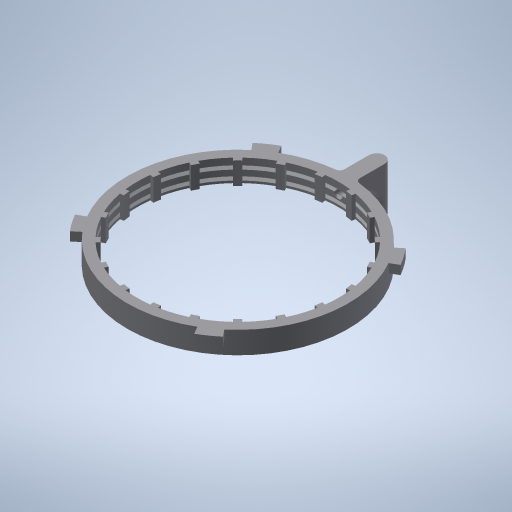
# Autodesk Inventor part: Sealing_ring_20x1_silicone_i
Saved by Autodesk Inventor 2023.2 (Build 272271000, 271)
## iProperties
Created: 2022-11-16
Part Number: Sealing_ring_20x1_silicone_i
Material: Generisch
Document SubType Name: Modeling
Designer: splath
Density: 1 g/cm^3
Appearance: Vorgabe
Author: splath
Autodesk Inventor part; units mm, degrees
ref_plane "Work Plane3" through (0, 0, 4) normal (0, 0, -1) x (0, -1, 0)
ref_plane "YZ Plane" through (0, 0, 0) normal (1, 0, 0) x (0, 1, 0)
sketch "Sketch1" plane through (0, 0, 0) normal (0, 1, 0) x (-1, 0, 0)
  line L0 (20.5, 5.8) -> (20.5, 4.7008) construction
  line L1 (22, 0) -> (25, 0)
  line L2 (25, 0) -> (25, 5)
  line L3 (25, 5) -> (22.8, 5)
  line L4 (21.5, 5) -> (21.5, 5.8) construction
  line L5 (21.5, 5.8) -> (20.5, 5.8) construction
  line L6 (0, -10.2759) -> (0, 12.2292) construction
  line L7 (30, 0) -> (-5, 0) construction
  line L8 (0, 9.0142) -> (16.75, 9.0142) construction
  line L9 (16.75, 9.0142) -> (16.75, -7.0609) construction
  line L10 (16.75, -7.0609) -> (0, -7.0609) construction
  line L11 (0, -7.0609) -> (0, 9.0142) construction
  line L12 (22, 0.2899) -> (22, 0)
  line L13 (23.3, 2.0523) -> (24.0071, 1.3452)
  line L14 (24.0071, 1.3452) -> (22.5, 0.2899)
  line L15 (22.5, 0.2899) -> (22, 0.2899)
  line L16 (20.5, 4.7008) -> (20.5, -3.6475) construction
  line L17 (22.8, 5) -> (22.8, 3.4859)
  line L18 (22.8, 2.6477) -> (24.0071, 3.4929)
  line L19 (24.0071, 3.4929) -> (23.3, 4.2)
  line L20 (23.3, 4.2) -> (22.8, 3.4859)
  line L21 (22.8, 1.3383) -> (23.3, 2.0523)
  line L22 (22.8, 5) -> (21.5, 5) construction
  line L23 (22.8, 3.4859) -> (22.8, 1.3383)
  line L24 (22.8, 0.5) -> (22.8, 0)
  point P0 (0, 0)
  dimension "d3" = 21.5
  dimension "d4" = 0.8
  dimension "d15" = 25
  dimension "d17" = 20.5
  dimension "d18" = 16.75
  dimension "d23" = 0.2899
  dimension "d24" = 5
  dimension "d70" = 22
  dimension "d72" = 1
  dimension "d102" = 22.8
  dimension "d104" = 80
  dimension "d106" = 0.5
  dimension "d107" = 80
  dimension "d121" = 0.5
  dimension "d122" = 0.5
  dimension "d123" = 0.5
  dimension "d124" = 45
  dimension "d125" = 0.8
  constraints: 46 end point, 12 perpendicular, 7 point on line, 6 parallel, 2 horizontal, 2 vertical, 2 other
  measures "d3" distance between parallel lines of L6 L4
  measures "d4" distance of L4.start L4.end
  measures "d15" distance between parallel lines of L6 L2
  measures "d17" distance between parallel lines of L6 L0
  measures "d18" distance of L9.end L10.end
  measures "d23" distance of L12.start L1.start
  measures "d24" distance of the line from the sketch origin of L3
  measures "d70" distance between parallel lines of L11 L12
  measures "d72" distance of L13.start L13.end
  measures "d102" distance from line of L3.end L11
  measures "d104" angle of L13 L14
  measures "d106" distance of L14.end L12.start
  measures "d107" angle of L13 L21
  measures "d121" distance of L24.start L24.end
  measures "d122" distance from line of L17 L19.end
  measures "d123" distance from line of L23 L13.start
  measures "d124" angle of L3 L19
  measures "d125" distance from line of L3 L19.end
revolve "Revolution1" add sketch "Sketch1" angle 360 about axis through (0, 0, -10) along (0, 0, 1) contours L24 L14 L13 L21 L23 L18 L19 L20 L17 L3 L2 L1
ref_plane "Work Plane2" through (0, 24.5, 2.5) normal (0, 1, 0) x (-1, 0, 0)
ref_plane "Work Plane1" through (0, 25, 2.5) normal (0, 1, 0) x (-1, 0, 0)
sketch "Sketch4" plane through (0, 24.5, 2.5) normal (0, 1, 0) x (-1, 0, 0)
  circle A0 centre (0, 0) radius 1.75
  circle A1 centre (0, 0) radius 0.9
  line L0 (0, 2.5) -> (0, -2.5) construction
  line L1 (25, -2.5) -> (-25, -2.5) construction
  point P0 (0, 0)
  dimension "d43" = 3.5
  dimension "d44" = 1.8
  dimension "d101" = 2.5
  constraints: 2 centre point, 2 coincident, 2 end point, 1 midpoint, 1 vertical
  measures "d43" diameter of A0
  measures "d44" diameter of A1
  measures "d101" distance from line of L1 A0.centre
extrude "Extrusion2" cut sketch "Sketch4" along normal blind 1 and the other way blind 5 contours A1
sketch "Sketch5" plane through (0, 0, 0) normal (1, 0, 0) x (0, 1, 0)
  line L0 (25, 0) -> (25, 5) construction
  line L1 (24.5, 13.7) -> (24.5, -8.7) construction
  line L2 (25, 0) -> (-25, 0) construction
  line L3 (24.5, 2.5) -> (25.5, 2.5)
  arc A0 (25.5, 2.5) -> (31.5, 8.5) centre (25.5, 8.5) ccw
  line L4 (31.5, 8.5) -> (31.5, 10.5)
  arc A1 (31.5, -3.5) -> (25.5, 2.5) centre (25.5, -3.5) ccw
  line L5 (31.5, -3.5) -> (31.5, -5.5)
  point P0 (0, 0)
  point P1 (28.721, 1.8909)
  point P2 (28.721, 3.1091)
  dimension "d23" = 0.2899
  dimension "d45" = 6
  dimension "d46" = 1
  dimension "d47" = 2
  constraints: 6 end point, 4 point on circle, 4 symmetric about line, 2 centre point, 2 tangent, 1 horizontal, 1 perpendicular, 1 other
  measures "d45" radius of A0
  measures "d46" distance of L3.start L3.end
  measures "d47" distance of L4.start L4.end
sweep "Sweep1" add profiles "Sketch4" path "Sketch5" path curves L3 A1 L5
sketch "Sketch3" plane through (0, 28.5, 4.5) normal (0, 1, 0) x (-1, 0, 0)
  line L0 (25, 0.5) -> (-25, 0.5) construction
  line L1 (25, -4.5) -> (-25, -4.5) construction
  line L2 (20.5, -3) -> (-20.5, -3) construction
  line L3 (20.5, -1) -> (-20.5, -1) construction
  line L4 (0, -1) -> (0, -3) construction
  point P0 (0, -4.5)
  point P1 (0, -2)
  point P2 (0, -2)
  constraints: 3 midpoint, 2 end point, 1 coincident
hole "Hole1" [suppressed]
sketch "Sketch8" plane through (0, 0, 5) normal (0, 0, -1) x (-1, 0, 0)
  line L0 (-1.75, 31.5) -> (1.75, 31.5)
  line L1 (1.75, 31.5) -> (1.75, 24.1443)
  line L2 (1.75, 24.1443) -> (-1.75, 24.1443)
  line L3 (-1.75, 24.1443) -> (-1.75, 31.5)
  line L4 (-1.75, 31.5) -> (-1.75, 25.5) construction
  line L5 (1.75, 31.5) -> (1.75, 25.5) construction
  arc A0 (1.75, 31.5) -> (-1.75, 31.5) centre (0, 31.5) ccw
  circle A1 centre (0, 31.5) radius 0.9 construction
  circle A2 centre (0, 31.5) radius 1.75 construction
  line L6 (1.75, 25.5) -> (-1.75, 25.5) construction
  point P0 (0, 0)
  point P1 (1.7253, 31.5)
  point P2 (-1.75, 31.5)
  constraints: 12 end point, 2 collinear, 2 parallel, 2 point on circle, 1 centre point, 1 coincident, 1 horizontal, 1 perpendicular, 1 tangent
extrude "Extrusion4" add sketch "Sketch8" along normal up to surface
fillet "Fillet1" radius 1 4 edges at (1.75, 24.9387, 3.75) (-1.75, 24.9387, 3.75) (1.75, 31.5, 0.75) (-1.75, 31.5, 0.75)
chamfer "Chamfer1" [suppressed]
sketch "Sketch9" plane through (0, 0, 5) normal (0, 0, 1) x (1, 0, 0)
  line L0 (0, -45.05) -> (0, 46.3) construction
  arc A0 (-4, -28) -> (4, -28) centre (0, -28) ccw
  line L1 (4, -28) -> (4, -24.6779)
  line L2 (-4, -28) -> (-4, -24.6779)
  arc A1 (-2.6442, 24.8598) -> (2.6442, 24.8598) centre (0, 0) ccw construction
  arc A2 (-4, -24.6779) -> (4, -24.6779) centre (0, 0) ccw
  arc A3 (13.5, -23.3827) -> (17.3553, -20.6832) centre (0, 0) ccw
  line L3 (13.5, -23.3827) -> (12.5, -21.6506)
  line L4 (17.3553, -20.6832) -> (16.0697, -19.1511)
  arc A4 (12.5, -21.6506) -> (16.0697, -19.1511) centre (0, 0) ccw
  point P0 (0, -25)
  point P1 (-25, 0)
  point P2 (0, -25)
  dimension "d77" = 8
  dimension "d78" = 3
  dimension "d94" = 27
  dimension "d95" = 10
  dimension "d96" = 30
  constraints: 13 point on circle, 10 end point, 4 centre point, 4 coincident, 4 point on line, 2 tangent, 1 vertical
  measures "d77" distance between parallel lines of L2 L1
  measures "d78" distance of point (0, -25) A0.centre
  measures "d94" radius of A3
  measures "d95" angle of L4 L3
  measures "d96" angle of L3 L0
extrude "Extrusion5" [suppressed]
extrude "Extrusion6" add sketch "Sketch9" against normal blind 2 contours L3 A4 L4 A3
sketch "Sketch10" plane through (0, -28, 5) normal (0, 0, 1) x (1, 0, 0)
  arc A0 (-4, 0) -> (4, 0) centre (0, 0) ccw construction
  point P0 (0, 28)
  constraints: 1 coincident
hole "Hole3" [suppressed]
sketch "Sketch12" plane through (0, 25.0079, 5) normal (0, 0, 1) x (0.6686669, -0.7435621, 0)
  line L0 (52.275, -47.0096) -> (-15.8624, 14.2647) construction
  line L1 (40.591, -16.3065) -> (41.4027, -16.2635)
  line L2 (41.4027, -16.2635) -> (41.3232, -14.7656)
  line L3 (41.3232, -14.7656) -> (40.5116, -14.8086)
  line L4 (40.591, -16.3065) -> (41.3232, -14.7656) construction
  line L5 (41.4027, -16.2635) -> (40.5116, -14.8086) construction
  circle A0 centre (18.595, -16.722) radius 22.8 construction
  arc A1 (40.591, -16.3065) -> (40.5116, -14.8086) centre (18.595, -16.722) ccw
  line L6 (40.9571, -15.536) -> (18.595, -16.722) construction
  dimension "d110" = 1.5
  dimension "d119" = 45
  dimension "d120" = 22
  constraints: 12 end point, 2 midpoint, 2 parallel, 2 point on circle, 1 centre point, 1 coincident, 1 perpendicular, 1 tangent
  measures "d110" distance of L3.end L1.start
  measures "d119" angle of L6 L0
  measures "d120" radius of A1
extrude "Extrusion8" add sketch "Sketch12" against normal up to surface (5 mm away)
pattern_circular "Circular Pattern1" count 4 over 360 about axis through (0, 0, 2.5) along (0, 0, 1) of "Extrusion6"
sketch "Sketch11" plane through (0, 0, 5) normal (0, 0, 1) x (0.9848078, -0.1736482, 0)
  circle A0 centre (0, 0) radius 21.5
  circle A1 centre (0, 0) radius 24
  dimension "d97" = 43
  dimension "d98" = 48
  constraints: 2 centre point, 2 coincident
  measures "d97" diameter of A0
  measures "d98" diameter of A1
sketch "Sketch6" plane through (0, 0, 4) normal (0, 0, -1) x (0, -1, 0)
  circle A0 centre (0, 0) radius 20.5 construction
  circle A1 centre (0, 0) radius 21.618
  dimension "d51" = 41.9365
  constraints: 1 centre point, 1 coincident
sketch "Sketch7" plane through (0, 0, 5.8) normal (0, 0, 1) x (1, 0, 0)
  circle A0 centre (0, 0) radius 20.5 construction
  constraints: 1 coincident
sketch "Sketch2" plane through (0, 0, 5) normal (0, 0, 1) x (1, 0, 0)
  circle A0 centre (0, 0) radius 25
  circle A1 centre (0, 0) radius 25 construction
  constraints: 1 centre point, 1 coincident, 1 concentric
pattern_circular "Circular Pattern2" count 20 over 360 about axis through (0, 0, 2.5) along (0, 0, 1) of "Extrusion8"
equation "\"d51\" = 2 * d17 + 2 * d50"
equation "\"d50\" = 0.468246"
body "Solid1"
